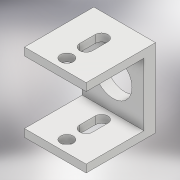
# Autodesk Inventor part: ShaftSyncAdapter
Saved by Autodesk Inventor 2018.2 (Build 222227000, 227)
## iProperties
Created: 2018-04-02
Part Number: ShaftSyncAdapter
Material: ABS Plastic
Document SubType Name: Modeling
Designer: Muchen He
Density: 1.06 g/cm^3
Appearance: Smooth - White
Author: Muchen He
Autodesk Inventor part; units mm, degrees
ref_plane "YZ Plane" through (0, 0, 0) normal (1, 0, 0) x (0, 1, 0)
ref_plane "XZ Plane" through (0, 0, 0) normal (0, 1, 0) x (-1, 0, 0)
ref_plane "XY Plane" through (0, 0, 0) normal (0, 0, 1) x (1, 0, 0)
sketch "Sketch1" plane through (0, 0, 0) normal (0, 1, 0) x (-1, 0, 0)
  circle A0 centre (0, 0) radius 4.9
  circle A1 centre (0, 0) radius 6.9
  line L0 (6.9, 8) -> (-5.9499, 8) construction
  line L1 (6.9, -8) -> (-5.9499, -8) construction
  line L2 (8, 8.15) -> (-8, 8.15)
  line L3 (-8, 8.15) -> (-8, -8.15)
  line L4 (-8, -8.15) -> (8, -8.15)
  line L5 (8, -8.15) -> (8, 8.15)
  line L6 (8, 8.15) -> (8, 10.15)
  line L7 (8, 10.15) -> (-8, 10.15)
  line L8 (-8, 10.15) -> (-8, 8.15)
  line L9 (-8, -8.15) -> (-8, -10.15)
  line L10 (-8, -10.15) -> (8, -10.15)
  line L11 (8, -10.15) -> (8, -8.15)
  point P0 (0, -8.15)
  dimension "d0" = 9.8
  dimension "d1" = 2
  dimension "d2" = 16
  dimension "d3" = 8
  dimension "d4" = 0.15
  dimension "d5" = 0.15
  dimension "d6" = 16
  dimension "d7" = 2
  dimension "d8" = 2
  constraints: 24 end point, 5 perpendicular, 3 horizontal, 2 centre point, 2 coincident, 2 parallel, 2 point on line, 1 midpoint, 1 vertical, 1 vertical alignment
  measures "d0" diameter of A0
  measures "d1" radial gap between concentric circles of A1 A0
  measures "d2" distance between parallel lines of L0 L1
  measures "d3" distance from line of point (0, 0) L0
  measures "d4" distance between parallel lines of L1 L4
  measures "d5" distance between parallel lines of L0 L2
  measures "d6" distance of L3.end L4.end
  measures "d7" distance of L2.start L6.end
  measures "d8" distance of L3.end L9.end
extrude "Extrusion1" add sketch "Sketch1" along normal blind 3 contours A1 | L5 L4 L3 L2 | L2 L8 L7 L6 | L11 L10 L9 L4
extrude "Extrusion2" add sketch "Sketch1" against normal blind 15 contours L2 L8 L7 L6 | L11 L10 L9 L4
sketch "Sketch2" plane through (-8, 3, 10.15) normal (0, 0, 1) x (1, 0, 0)
  circle A0 centre (8, -15) radius 1.65
  line L0 (16, -18) -> (0, -18) projected
  point P0 (8, -3)
  point P1 (8, -18)
  dimension "d13" = 3.3
  dimension "d14" = 3
  constraints: 1 centre point, 1 midpoint, 1 vertical alignment
  measures "d13" diameter of A0
  measures "d14" distance from line of L0 A0.centre
extrude "Extrusion3" cut sketch "Sketch2" against normal through all
sketch "Sketch3" plane through (-8, 3, 10.15) normal (0, 0, 1) x (1, 0, 0)
  line L0 (8, -10) -> (8, -6) construction
  line L1 (9.65, -10) -> (9.65, -6)
  line L2 (6.35, -6) -> (6.35, -10)
  arc A0 (6.35, -10) -> (9.65, -10) centre (8, -10) ccw
  arc A1 (9.65, -6) -> (6.35, -6) centre (8, -6) ccw
  circle A2 centre (8, -15) radius 1.65 projected
  point P0 (8, -3)
  point P1 (8, -8)
  dimension "d17" = 3.3
  dimension "d18" = 4
  dimension "d19" = 5
  constraints: 8 end point, 4 point on circle, 4 tangent, 2 centre point, 1 midpoint, 1 parallel, 1 vertical, 1 vertical alignment
  measures "d17" distance between parallel lines of L2 L1
  measures "d18" distance of L0.start L0.end
  measures "d19" distance of A2.centre L0.start
extrude "Extrusion4" cut sketch "Sketch3" against normal through all contours A0 L2 A1 L1
body "Solid1"
